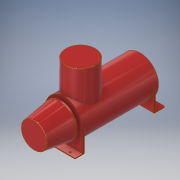
# Autodesk Inventor part: Compressor_PX06
Saved by Autodesk Inventor 2018 (Build 220112000, 112)
## iProperties
Created: 2017-11-21
Part Number: Compressor_PX06
Material: Polyethylene, High Density
Document SubType Name: Modeling
Designer: P136265
Density: 0.952 g/cm^3
Appearance: Smooth - Off-White
Mass: 2273.74 g
Surface Area: 1454.95 cm^2
Volume: 2388.38 cm^3
Author: P136265
Autodesk Inventor part; units mm, degrees
ref_plane "YZ Plane" through (0, 0, 0) normal (1, 0, 0) x (0, 1, 0)
sketch "Sketch1" plane through (0, 0, 0) normal (0, 0, 1) x (1, 0, 0)
  circle A0 centre (0, 0) radius 50
  dimension "d0" = 100
  constraints: 1 centre point, 1 coincident
  measures "d0" diameter of A0
extrude "Extrusion1" add sketch "Sketch1" along normal blind 205
sketch "Sketch2" plane through (0, 0, 0) normal (1, 0, 0) x (0, 1, 0)
  line L0 (-50, 0) -> (50, 0) construction
  line L1 (0, 0) -> (0, -80)
  line L2 (0, -80) -> (35, -80)
  line L3 (0, 0) -> (5, 0)
  line L4 (5, 0) -> (5, -3.5)
  line L5 (9, -7.5) -> (45, -7.5)
  line L6 (45, -7.5) -> (45, -12.5)
  line L7 (45, -12.5) -> (35, -80)
  arc A0 (5, -3.5) -> (9, -7.5) centre (9, -3.5) ccw
  point P0 (5, -7.5)
  dimension "d3" = 80
  dimension "d4" = 35
  dimension "d5" = 5
  dimension "d6" = 7.5
  dimension "d7" = 40
  dimension "d8" = 5
  dimension "d9" = 4
  constraints: 14 end point, 3 perpendicular, 3 point on line, 2 point on circle, 2 tangent, 2 vertical, 1 centre point
  measures "d3" distance of L1.start L1.end
  measures "d4" distance of L1.end L2.end
  measures "d5" distance of L1.start L3.end
  measures "d6" distance of L3.end point (5, -7.5)
  measures "d7" distance of point (5, -7.5) L5.end
  measures "d8" distance of L5.end L6.end
  measures "d9" radius of A0
revolve "Revolution1" add sketch "Sketch2" angle 360 about axis through (0, 0, 0) along (0, 0, -1)
ref_plane "Work Plane1" through (0, 120, 0) normal (0, 1, 0) x (-1, 0, 0)
sketch "Sketch3" plane through (0, 120, 0) normal (0, 1, 0) x (-1, 0, 0)
  line L0 (-50, 0) -> (50, 0) construction
  circle A0 centre (0, 45) radius 40
  line L1 (-50, 0) -> (-50, 205) construction
  point P0 (0, 0)
  dimension "d19" = 80
  dimension "d20" = 45
  dimension "d21" = 50
  constraints: 1 centre point
  measures "d19" diameter of A0
  measures "d20" distance of point (0, 0) A0.centre
  measures "d21" distance from line of L1 A0.centre
extrude "Extrusion2" add sketch "Sketch3" against normal blind 90
ref_plane "Work Plane2" through (0, 0, 195) normal (0, 0, 1) x (1, 0, 0)
sketch "Sketch4" plane through (0, 0, 195) normal (0, 0, 1) x (1, 0, 0)
  circle A0 centre (0, -60) radius 50 construction
  circle A1 centre (0, 0) radius 45 construction
  arc A2 (-44.9972, -0.4998) -> (44.9999, 0.1033) centre (0.0033, -0.4998) ccw
  line L0 (-50, -60) -> (50, -60)
  circle A3 centre (0, 0) radius 50 construction
  line L1 (-50, -60) -> (-50, 0)
  circle A4 centre (0, 0) radius 50 construction
  line L2 (50, -60) -> (50, 0)
  arc A5 (-50, 0) -> (50, 0) centre (0, 0) ccw
  point P0 (-44.9972, -38.1998)
  point P1 (44.9999, -81.7947)
  dimension "d26" = 100
  dimension "d27" = 60
  dimension "d29" = 90
  constraints: 10 point on circle, 6 end point, 4 centre point, 2 horizontal alignment, 2 tangent, 1 coincident, 1 horizontal, 1 parallel, 1 vertical, 1 vertical alignment, 2 other
  measures "d26" diameter of A0
  measures "d27" distance of point (0, 0) A0.centre
  measures "d29" diameter of A1
extrude "Extrusion3" add sketch "Sketch4" against normal blind 5
sketch "Sketch7" plane through (0, 0, 0) normal (0, 0, -1) x (-1, 0, 0)
  line L0 (-50, -60) -> (50, -60) construction
  line L1 (50, -60) -> (50, 0) construction
  arc A0 (-50, 0) -> (50, 0) centre (0, 0) ccw construction
  line L2 (-50, 0) -> (-50, -60) construction
  line L3 (-50, -60) -> (50, -60)
  line L4 (50, -60) -> (50, 0)
  circle A1 centre (0, 0) radius 50 construction
  line L5 (-50, -60) -> (50, -60) projected
  line L6 (-50, 0) -> (-50, -60) projected
  line L7 (-50, -60) -> (-50, 0)
  arc A2 (-50, 0) -> (50, 0) centre (0, 0) ccw
  constraints: 6 end point, 3 tangent, 2 point on circle, 1 centre point, 1 collinear, 1 horizontal, 1 perpendicular
extrude "Extrusion5" add sketch "Sketch7" against normal blind 5
sketch "Sketch8" plane through (0, 0, 0) normal (0, 0, -1) x (-1, 0, 0)
  line L0 (50, -60) -> (-50, -60) projected
  line L1 (50, 0) -> (50, -60) construction
  line L2 (-50, -60) -> (50, -60)
  line L3 (50, -60) -> (50, -57.5)
  line L4 (50, -57.5) -> (-50, -57.5)
  line L5 (-50, -57.5) -> (-50, -60)
  point P0 (0, 0)
  dimension "d37" = 2.5
  constraints: 8 end point, 2 parallel, 1 horizontal, 1 perpendicular, 1 point on line
  measures "d37" distance of L3.end L2.end
extrude "Extrusion6" add sketch "Sketch8" along normal blind 20
sketch "Sketch9" plane through (-50, -57.5, 0) normal (0, 1, 0) x (1, 0, 0)
  circle A0 centre (20, 12.5) radius 5 construction
  circle A1 centre (80, 12.5) radius 5 construction
  line L0 (0, 0) -> (0, 20) construction
  line L1 (100, 0) -> (0, 0) construction
  point P0 (50, 0)
  dimension "d40" = 10
  dimension "d41" = 10
  dimension "d42" = 60
  dimension "d43" = 20
  dimension "d45" = 12.5
  constraints: 2 centre point, 1 horizontal alignment
  measures "d40" diameter of A0
  measures "d41" diameter of A1
  measures "d42" distance of A0.centre A1.centre
  measures "d43" distance from line of L0 A0.centre
  measures "d45" distance from line of L1 A0.centre
hole "Hole1" at (-30, -57.5, -12.5) at (30, -57.5, -12.5) direction (0, -1, 0) diameter 5 end through all
sketch "Sketch10" plane through (0, 0, 195) normal (0, 0, 1) x (1, 0, 0)
  line L0 (50, 0) -> (50, -60) construction
  line L1 (-50, -60) -> (50, -60)
  line L2 (50, -60) -> (50, -57.5)
  line L3 (50, -57.5) -> (-50, -57.5)
  line L4 (-50, -57.5) -> (-50, -60)
  point P0 (0, 0)
  dimension "d53" = 2.5
  constraints: 8 end point, 2 parallel, 1 horizontal, 1 perpendicular, 1 point on line
  measures "d53" distance of L2.end L1.end
extrude "Extrusion7" add sketch "Sketch10" along normal blind 25
sketch "Sketch11" plane through (-50, -57.5, 195) normal (0, 1, 0) x (1, 0, 0)
  circle A0 centre (20, -17.5) radius 5 construction
  circle A1 centre (80, -17.5) radius 5 construction
  line L0 (100, -25) -> (0, -25) construction
  line L1 (0, 0) -> (0, -25) construction
  point P0 (50, 195)
  dimension "d56" = 10
  dimension "d57" = 10
  dimension "d58" = 7.5
  dimension "d59" = 20
  dimension "d60" = 60
  constraints: 2 centre point, 1 horizontal alignment
  measures "d56" diameter of A0
  measures "d57" diameter of A1
  measures "d58" distance from line of L0 A1.centre
  measures "d59" distance from line of L1 A0.centre
  measures "d60" distance of A1.centre A0.centre
hole "Hole2" at (-30, -57.5, 212.5) at (30, -57.5, 212.5) direction (0, -1, 0) diameter 5 end through all
fillet "Fillet1" radius 2 9 edges at (-50, 0, 205) (-50, -58.75, 220) (50, -58.75, 220) (-50, -58.75, -20) (50, -58.75, -20) (0, -60, 5) (0, -60, 190) (0, -35, -80) (40, 120, 45)
body "Solid1"
